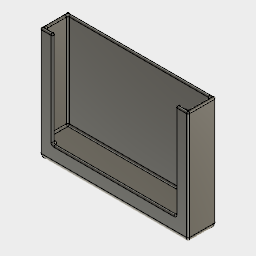
TelepresenceSleeve (Autodesk Fusion 360 design; units mm, degrees)
Autodesk Fusion 360 part; units mm, degrees
sketch "Sketch1" plane through (0, 0, 0) normal (0, 0, 1) x (1, 0, 0)
  line L0 (37.25, -5.75) -> (-37.25, -5.75)
  line L1 (-37.25, -5.75) -> (-37.25, 5.75)
  line L2 (-37.25, 5.75) -> (37.25, 5.75)
  line L3 (37.25, 5.75) -> (37.25, -5.75)
  line L4 (37.25, -5.75) -> (-37.25, 5.75) construction
  line L5 (-37.25, -5.75) -> (37.25, 5.75) construction
  line L6 (38.85, -7.35) -> (-38.85, -7.35)
  line L7 (-38.85, -7.35) -> (-38.85, 7.35)
  line L8 (-38.85, 7.35) -> (38.85, 7.35)
  line L9 (38.85, 7.35) -> (38.85, -7.35)
  line L10 (38.85, -7.35) -> (-38.85, 7.35) construction
  line L11 (-38.85, -7.35) -> (38.85, 7.35) construction
  line L12 (0, 0) -> (0, -13) construction
  line L13 (-32.25, -5.75) -> (-32.25, -7.35)
  line L14 (32.25, -5.75) -> (32.25, -7.35)
  line L15 (-2.0248, -1.55) -> (2.0248, -1.55)
  line L16 (2.0248, 1.55) -> (-2.0248, 1.55)
  line L17 (-2.0248, -1.55) -> (-2.0248, 1.55) construction
  arc A0 (-2.0248, 1.55) -> (-2.0248, -1.55) centre (0, 0) ccw
  arc A1 (2.0248, -1.55) -> (2.0248, 1.55) centre (0, 0) ccw
  point P0 (-2.0248, 0)
  dimension "d1" = 74.5
  dimension "d2" = 11.5
  dimension "d3" = 77.7
  dimension "d4" = 14.7
  dimension "d5" = 32.25
  dimension "d6" = 32.25
  dimension "d11" = 5.1
  dimension "d26" = 3.1
  measures "d1" distance of L1.end L2.end
  measures "d2" distance of L0.end L1.end
  measures "d3" distance of L7.end L8.end
  measures "d4" distance of L6.end L7.end
  measures "d5" distance of L12 L13
  measures "d6" distance of L12 L14
  measures "d11" diameter of A0
  measures "d26" distance of L15.start L16.end
extrude "Extrude1" add sketch "Sketch1" along normal blind 10 contours L0 L1 L2 L3 L6 L7 L8 L9 L13 L14 | L0 L1 L2 L3 | L0 L6 L13 L14 | L15 L16 A0 A1
extrude "Extrude2" add sketch "Sketch1" along normal blind 60 contours L0 L1 L2 L3 L6 L7 L8 L9 L13 L14
extrude "Extrude3" cut sketch "Sketch1" along normal blind 9 contours L15 L16 A0 A1
sketch "Sketch3" plane through (0, 7.35, 0) normal (0, 1, 0) x (-1, 0, 0)
  line L0 (-38.85, 0) -> (38.85, 0)
  line L1 (38.85, 0) -> (38.85, 60)
  line L2 (38.85, 60) -> (-38.85, 60)
  line L3 (-38.85, 60) -> (-38.85, 0)
  line L4 (0, 0) -> (0, 3) construction
  circle A0 centre (0, 3) radius 1.25
  dimension "d14" = 3
  dimension "d15" = 2.5
  measures "d14" distance of L4.start L4.end
  measures "d15" diameter of A0
fillet "Fillet1" radius 0.79 32 edges at (-32.25, -7.35, 35) (-32.25, -5.75, 35) (0, -7.35, 10) (-32.25, -6.55, 60) (-35.55, -7.35, 60) (-34.75, -5.75, 60) (-37.25, 0, 60) (-38.85, 0, 60) (0, 7.35, 60) (0, 5.75, 60) (38.85, 0, 60) (37.25, 0, 60) (34.75, -5.75, 60) (32.25, -6.55, 60) (35.55, -7.35, 60) (32.25, -7.35, 35) (38.85, -7.35, 30) (38.85, 7.35, 30) (32.25, -5.75, 35) (37.25, 5.75, 35) (-37.25, -5.75, 35) (37.25, -5.75, 35) (-37.25, 5.75, 35) (-34.75, -5.75, 10) (-37.25, 0, 10) (0, 5.75, 10) (37.25, 0, 10) (34.75, -5.75, 10) (32.25, -6.55, 10) (-32.25, -6.55, 10) (-38.85, 7.35, 30) (-38.85, -7.35, 30)
fillet "Fillet2" radius 3 8 edges at (-38.85, 0, 0) (-38.6186, -7.1186, 0) (0, -7.35, 0) (38.6186, -7.1186, 0) (38.85, 0, 0) (38.6186, 7.1186, 0) (0, 7.35, 0) (-38.6186, 7.1186, 0)
extrude "Extrude4" cut sketch "Sketch3" against normal blind 7 draft -2 contours A0
fillet "Fillet3" radius 0.7 2 edges at (0, 7.35, 4.25) (0, 7.0815, 1.7594)
equation "d3 = d1 + ( 1.6 * 2 ) * 1 mm"
equation "d4 = d2 + ( 1.6 * 2 ) * 1 mm"
equation "d5 = ( d1 / 2 ) - 5 mm"
equation "d6 = d5"
named bodies: "PhoneHolder"
